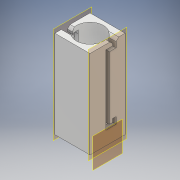
# Autodesk Inventor part: RescueKitThrow_pipe
Saved by Autodesk Inventor 2018.3 (Build 223284000, 284)
## iProperties
Created: 2019-02-10
Part Number: RescueKitThrow_pipe
Material: ABS プラスチック
Document SubType Name: Modeling
Designer: shun2
Density: 1.06 g/cm^3
Appearance: 滑らか - 白
Author: shun2
Autodesk Inventor part; units mm, degrees
ref_plane "YZ Plane" through (0, 0, 0) normal (1, 0, 0) x (0, 1, 0)
ref_plane "XZ Plane" through (0, 0, 0) normal (0, 1, 0) x (-1, 0, 0)
ref_plane "XY Plane" through (0, 0, 0) normal (0, 0, 1) x (1, 0, 0)
sketch "スケッチ1" plane through (0, 0, 0) normal (0, 0, 1) x (1, 0, 0)
  circle A0 centre (0, 0) radius 0.6
  line L0 (-0.6, 0) -> (0.6, 0)
  line L1 (-0.6, 0) -> (0.6, 0)
  line L2 (-13, 13) -> (13, 13)
  line L3 (13, 13) -> (13, -13)
  line L4 (13, -13) -> (-13, -13)
  line L5 (-13, -13) -> (-13, 13)
  dimension "d1" = 1.2
  dimension "d57" = 26
  dimension "d58" = 26
  constraints: 12 end point, 3 horizontal, 2 parallel, 2 point on circle, 1 centre point, 1 perpendicular
  measures "d1" diameter of A0
  measures "d57" distance of L3.end L4.end
  measures "d58" distance of L2.end L3.end
extrude "押し出し1" add sketch "スケッチ1" along normal blind 5
sketch "スケッチ2" plane through (0, 0, 5) normal (0, 0, 1) x (1, 0, 0)
  circle A0 centre (0, 0) radius 0.6 projected
  circle A1 centre (0, 0) radius 10
  line L0 (-0.6, 0) -> (0.6, 0)
  line L1 (13, 0) -> (13, 13)
  line L2 (-0.6, 0) -> (0.6, 0)
  line L3 (-13, 13) -> (13, 13)
  line L4 (13, 13) -> (13, -13)
  line L5 (13, -13) -> (-13, -13)
  line L6 (-13, -13) -> (-13, 13)
  dimension "d5" = 20
  dimension "d59" = 26
  dimension "d60" = 26
  constraints: 14 end point, 3 horizontal, 2 parallel, 2 perpendicular, 2 point on circle, 1 centre point, 1 coincident
  measures "d5" diameter of A1
  measures "d59" distance of L4.end L5.end
  measures "d60" distance of L3.end L4.end
extrude "押し出し2" add sketch "スケッチ2" along normal blind 60 contours L4 L5 L6 L3 L1
ref_plane "作業平面3" through (13, -13, 0) normal (1, 0, 0) x (0, 0, -1)
ref_plane "作業平面4" through (13, 0, 0) normal (1, 0, 0) x (0, 1, 0)
sketch "スケッチ3" plane through (13, 0, 0) normal (1, 0, 0) x (0, 1, 0)
  line L0 (-13, 0) -> (13, 0) projected
  line L1 (-13, 0) -> (-13, 65) projected
  line L2 (1.25, 59) -> (-1.25, 59)
  line L3 (-1.25, 59) -> (-1.25, 10)
  line L4 (-1.25, 10) -> (1.25, 10)
  line L5 (1.25, 10) -> (1.25, 59)
  point P0 (0, 0)
  point P1 (0, 0)
  point P2 (0, 0)
  point P3 (0, 59)
  dimension "d39" = 2.5
  dimension "d40" = 49
  constraints: 8 end point, 2 parallel, 1 horizontal, 1 perpendicular, 1 other
  measures "d39" distance of L4.end L3.end
  measures "d40" distance of L3.end L2.end
extrude "押し出し3" cut sketch "スケッチ3" against normal blind 30
ref_plane "作業平面5" through (13, 0, 0) normal (1, 0, 0) x (0, 1, 0)
sketch "スケッチ4" plane through (13, 0, 0) normal (1, 0, 0) x (0, 1, 0)
  line L0 (-1.25, 59) -> (1.25, 59) projected
  line L1 (-1.25, 59) -> (6.25, 59)
  line L2 (6.25, 59) -> (6.25, 61.5)
  line L3 (3.75, 61.5) -> (-1.25, 61.5)
  line L4 (-1.25, 61.5) -> (-1.25, 59)
  line L5 (6.25, 59) -> (3.75, 59)
  line L6 (3.75, 61.5) -> (3.75, 66.5)
  line L7 (3.75, 66.5) -> (6.25, 66.5)
  line L8 (6.25, 66.5) -> (6.25, 59)
  line L9 (-1.25, 10) -> (6.25, 10)
  line L10 (6.25, 10) -> (6.25, 12.5)
  line L11 (3.75, 12.5) -> (-1.25, 12.5)
  line L12 (-1.25, 12.5) -> (-1.25, 10)
  line L13 (6.25, 10) -> (3.75, 10)
  line L14 (3.75, 12.5) -> (3.75, 15)
  line L15 (3.75, 15) -> (6.25, 15)
  line L16 (6.25, 15) -> (6.25, 10)
  point P0 (0, 0)
  point P1 (-1, 10)
  dimension "d49" = 7.5
  dimension "d50" = 2.5
  dimension "d51" = 2.5
  dimension "d52" = 7.5
  dimension "d53" = 7.5
  dimension "d54" = 2.5
  dimension "d55" = 2.5
  dimension "d56" = 5
  constraints: 32 end point, 8 parallel, 4 horizontal, 4 perpendicular
  measures "d49" distance of L3.end L2.end
  measures "d50" distance of L2.end L1.end
  measures "d51" distance of L6.end L7.end
  measures "d52" distance of L5.end L6.end
  measures "d53" distance of L11.end L10.end
  measures "d54" distance of L10.end L9.end
  measures "d55" distance of L14.end L15.end
  measures "d56" distance of L13.end L14.end
extrude "押し出し4" cut sketch "スケッチ4" against normal blind 8
ref_plane "作業平面2" through (-13, 0, 0) normal (1, 0, 0) x (0, 1, 0)
sketch "スケッチ5" plane through (-13, 0, 0) normal (1, 0, 0) x (0, 1, 0)
  line L0 (5, 10) -> (5, 10) projected
  line L1 (1.2591, 59) -> (-6.2409, 59)
  line L2 (-6.2409, 59) -> (-6.2409, 61.5)
  line L3 (-3.7409, 61.5) -> (1.2591, 61.5)
  line L4 (1.2591, 61.5) -> (1.2591, 59)
  line L5 (-6.2409, 59) -> (-3.7409, 59)
  line L6 (-3.7409, 61.5) -> (-3.7409, 66.5)
  line L7 (-3.7409, 66.5) -> (-6.2409, 66.5)
  line L8 (-6.2409, 66.5) -> (-6.2409, 59)
  line L9 (1.2591, 10) -> (-6.2409, 10)
  line L10 (-6.2409, 10) -> (-6.2409, 12.5)
  line L11 (-3.7409, 12.5) -> (1.2591, 12.5)
  line L12 (1.2591, 12.5) -> (1.2591, 10)
  line L13 (-6.2409, 10) -> (-3.7409, 10)
  line L14 (-3.7409, 12.5) -> (-3.7409, 15)
  line L15 (-3.7409, 15) -> (-6.2409, 15)
  line L16 (-6.2409, 15) -> (-6.2409, 10)
  point P0 (0, 0)
  point P1 (0.4791, 10)
  point P2 (1, 59)
  dimension "d41" = 7.5
  dimension "d42" = 2.5
  dimension "d43" = 2.5
  dimension "d44" = 7.5
  dimension "d45" = 7.5
  dimension "d46" = 2.5
  dimension "d47" = 2.5
  dimension "d48" = 5
  constraints: 32 end point, 8 parallel, 4 horizontal, 4 perpendicular, 1 horizontal alignment, 1 other
  measures "d41" distance of L2.end L3.end
  measures "d42" distance of L1.end L2.end
  measures "d43" distance of L7.end L6.end
  measures "d44" distance of L6.end L5.end
  measures "d45" distance of L10.end L11.end
  measures "d46" distance of L9.end L10.end
  measures "d47" distance of L15.end L14.end
  measures "d48" distance of L14.end L13.end
extrude "押し出し5" cut sketch "スケッチ5" along normal blind 8
chamfer "面取り2" distance 2 angle 45 4 edges at (-11.137, -3.7409, 65) (-10.4067, -6.2409, 65) (10.4031, 6.25, 65) (11.1351, 3.75, 65)
